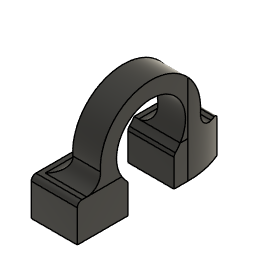
56b14100-354a-432f-bf98-abde912a1bf3 (Autodesk Fusion 360 design; units mm, degrees)
Autodesk Fusion 360 part; units mm, degrees
sketch "Esboço1" plane through (0, 0, -10.4303) normal (0, 0, 1) x (-1, 0, 0)
  line L0 (29.155, -19.6424) -> (-29.155, -19.6424)
  line L1 (-29.155, -19.6424) -> (-29.155, 12.3576)
  line L2 (-29.155, 12.3576) -> (29.155, 12.3576)
  line L3 (29.155, 12.3576) -> (29.155, -19.6424)
  circle A0 centre (-25.5, 38.3576) radius 3.95
  line L4 (15.7, 44.8576) -> (15.7, 39.0576)
  line L5 (15.7, 39.0576) -> (-15.7, 39.0576)
  line L6 (-15.7, 39.0576) -> (-15.7, 44.8576)
  line L7 (-15.7, 44.8576) -> (15.7, 44.8576)
  circle A1 centre (25.5, 38.3576) radius 3.95
  line L8 (11.25, -25.6424) -> (12.25, -26.6424)
  line L9 (12.25, -26.6424) -> (12.25, -34.1424)
  line L10 (12.25, -34.1424) -> (9.75, -34.1424)
  line L11 (9.75, -34.1424) -> (9.75, -45.1424)
  line L12 (9.75, -45.1424) -> (12.25, -45.1424)
  line L13 (12.25, -45.1424) -> (12.25, -52.6424)
  line L14 (12.25, -52.6424) -> (11.25, -53.6424)
  line L15 (11.25, -53.6424) -> (18, -53.6424)
  arc A2 (18, -53.6424) -> (28, -43.6424) centre (18, -43.6424) ccw
  line L16 (28, -43.6424) -> (28, -25.6424)
  line L17 (28, -25.6424) -> (38.8944, -20.1952)
  arc A3 (38.8944, -20.1952) -> (40, -18.4064) centre (38, -18.4064) ccw
  line L18 (40, -18.4064) -> (40, 11.1215)
  arc A4 (40, 11.1215) -> (38.8944, 12.9103) centre (38, 11.1215) ccw
  line L19 (38.8944, 12.9103) -> (32.2111, 16.252)
  arc A5 (32.2111, 16.252) -> (30.8695, 16.5687) centre (30.8695, 13.5687) ccw
  line L20 (30.8695, 16.5687) -> (28.9711, 16.5687)
  arc A6 (27.2503, 17.1112) -> (28.9711, 16.5687) centre (28.9711, 19.5687) ccw
  line L21 (27.2503, 17.1112) -> (22.237, 20.6216)
  arc A7 (21.5003, 24.7998) -> (22.237, 20.6216) centre (23.9577, 23.0791) ccw
  line L22 (21.5003, 24.7998) -> (29.1862, 35.7765)
  arc A8 (29.1862, 35.7765) -> (27.6041, 42.3354) centre (25.5, 38.3576) ccw
  line L23 (27.6041, 42.3354) -> (20.6582, 46.0094)
  arc A9 (20.6582, 46.0094) -> (19.2554, 46.3576) centre (19.2554, 43.3576) ccw
  line L24 (19.2554, 46.3576) -> (-19.2554, 46.3576)
  arc A10 (-19.2554, 46.3576) -> (-20.6582, 46.0094) centre (-19.2554, 43.3576) ccw
  line L25 (-20.6582, 46.0094) -> (-27.6041, 42.3354)
  arc A11 (-27.6041, 42.3354) -> (-29.1862, 35.7765) centre (-25.5, 38.3576) ccw
  line L26 (-29.1862, 35.7765) -> (-21.5003, 24.7998)
  arc A12 (-22.237, 20.6216) -> (-21.5003, 24.7998) centre (-23.9577, 23.0791) ccw
  line L27 (-22.237, 20.6216) -> (-27.2503, 17.1112)
  arc A13 (-28.9711, 16.5687) -> (-27.2503, 17.1112) centre (-28.9711, 19.5687) ccw
  line L28 (-28.9711, 16.5687) -> (-30.8695, 16.5687)
  arc A14 (-30.8695, 16.5687) -> (-32.2111, 16.252) centre (-30.8695, 13.5687) ccw
  line L29 (-32.2111, 16.252) -> (-38.8944, 12.9103)
  arc A15 (-38.8944, 12.9103) -> (-40, 11.1215) centre (-38, 11.1215) ccw
  line L30 (-40, 11.1215) -> (-40, -18.4064)
  arc A16 (-40, -18.4064) -> (-38.8944, -20.1952) centre (-38, -18.4064) ccw
  line L31 (-38.8944, -20.1952) -> (-28, -25.6424)
  line L32 (-28, -25.6424) -> (-28, -43.6424)
  arc A17 (-28, -43.6424) -> (-18, -53.6424) centre (-18, -43.6424) ccw
  line L33 (-18, -53.6424) -> (-11.25, -53.6424)
  line L34 (-11.25, -53.6424) -> (-12.25, -52.6424)
  line L35 (-12.25, -52.6424) -> (-12.25, -45.1424)
  line L36 (-12.25, -45.1424) -> (-9.75, -45.1424)
  line L37 (-9.75, -45.1424) -> (-9.75, -34.1424)
  line L38 (-9.75, -34.1424) -> (-12.25, -34.1424)
  line L39 (-12.25, -34.1424) -> (-12.25, -26.6424)
  line L40 (-12.25, -26.6424) -> (-11.25, -25.6424)
  line L41 (-11.25, -25.6424) -> (11.25, -25.6424)
  line L42 (-28, -31.6424) -> (-23, -31.6424)
  line L43 (-23, -31.6424) -> (-23, -47.6424)
  line L44 (-23, -47.6424) -> (-28, -47.6424)
  line L45 (-28, -47.6424) -> (-28, -31.6424)
  line L46 (-23, -39.6424) -> (-28, -39.6424) construction
  line L47 (-28, -41.6424) -> (-23, -41.6424)
  line L48 (-28, -37.6424) -> (-23, -37.6424)
  line L49 (-28, -31.6424, 0) -> (-28, -31.6424, 3.5)
  line L50 (-28, -47.6424, 3.5) -> (-28, -47.6424, 0)
  line L51 (-28, -39.6424, 0) -> (-28, -39.6424, 12) construction
  line L52 (-28, -31.6424, 0) -> (-28, -31.6424, 2.5)
  arc A18 through (-28, -34.1565, 5.6071) (-28, -39.6424, 11.5) (-28, -45.1284, 5.6071)
  line L53 (-28, -46.6246, 4) -> (-28, -47.1424, 4)
  line L54 (-28, -32.1424, 4) -> (-28, -32.6603, 4)
  arc A19 through (-28, -34.1565, 5.6071) (-28, -33.7582, 4.4779) (-28, -32.6603, 4)
  arc A20 through (-28, -45.1284, 5.6071) (-28, -45.5267, 4.4779) (-28, -46.6246, 4)
  arc A21 through (-28, -31.6424, 3.5) (-28, -31.7889, 3.8536) (-28, -32.1424, 4)
  arc A22 through (-28, -47.6424, 3.5) (-28, -47.496, 3.8536) (-28, -47.1424, 4)
  line L55 (-28, -37.1424, 0) -> (-28, -37.1424, 2.9896)
  line L56 (-28, -42.1424, 0) -> (-28, -42.1424, 2.9896)
  arc A23 through (-28, -36.9954, 3.3438) (-28, -39.6424, 9.75) (-28, -42.2895, 3.3438)
  arc A24 through (-28, -36.9954, 3.3438) (-28, -37.1042, 3.1813) (-28, -37.1424, 2.9896)
  arc A25 through (-28, -42.2895, 3.3438) (-28, -42.1807, 3.1813) (-28, -42.1424, 2.9896)
  line L57 (-28, -32.1424, 4) -> (-28, -36.4703, 4)
  line L58 (-28, -42.8146, 4) -> (-28, -47.1424, 4)
  line L59 (-23, -44.6424) -> (-28, -44.6424) construction
  line L60 (-23, -34.6424) -> (-28, -34.6424) construction
  circle A26 centre (-25.5, -34.6424) radius 1
  circle A27 centre (-25.5, -44.6424) radius 1
  dimension "d199" = 2
  dimension "d200" = 2
  dimension "d201" = 8
  dimension "d202" = 8
  dimension "d205" = 6
  dimension "d206" = 7.5
  dimension "d207" = 2.5
  dimension "d208" = 11
  dimension "d209" = 1.5
  dimension "d210" = 0.5
  dimension "d211" = 2.5
  dimension "d212" = 2.5
  dimension "d213" = 0.5
  dimension "d222" = 5
  dimension "d223" = 5
  dimension "d225" = 2
  dimension "d228" = 4
  constraint horizontal L42
  constraint vertical L43
  constraint horizontal L44
  constraint vertical L45
  constraint coincident L32 L42.start
  constraint coincident L32 L46.end
  constraint perpendicular L32 L46
  constraint coincident L43 L46.start
  constraint coincident L45 L47.start
  constraint coincident L43 L47.end
  constraint perpendicular L43 L47
  constraint coincident L45 L48.start
  constraint coincident L43 L48.end
  constraint perpendicular L43 L48
  constraint coincident L43 L59.start
  constraint coincident L45 L59.end
  constraint perpendicular L45 L59
  constraint coincident L43 L60.start
  constraint coincident L45 L60.end
  constraint parallel L48 L60
  constraint midpoint L60 A26.centre
  constraint midpoint L59 A27.centre
  constraint equal A26 A27
  measures "d199" distance of L46 L47
  measures "d200" distance of L46 L48
  measures "d201" distance of L42 L46
  measures "d202" distance of L44 L46
  measures "d205" distance of L45 L46.end
  measures "d207" distance of L42.start L45.end
  measures "d222" distance of L46 L59
  measures "d223" distance of L46 L60
  measures "d225" diameter of A27
extrude "Extrusão1" add sketch "Esboço1" along normal blind 5 contours L32 L45 L49 L52 L54 A21 L55 A23 A24 L57 | L32 L45 L50 L53 A22 L56 A23 A25 L58 in plane through (28, 0, -10.4303) normal (-1, 0, 0) makes body 1 at (26.3333, 33.4758, -10.4303) makes body 2 at (26.3333, 43.9758, -10.4303)
extrude "Extrusão2" add sketch "Esboço1" along normal blind 3 contours A18 A19 A20 A23 L57 L58 in plane through (28, 0, -10.4303) normal (-1, 0, 0) bodies 1 2
fillet "Arredondamento1" radius 1.5 2 edges at (25, 34.5653, -6.4303) (25, 44.7196, -6.4303) on bodies 1
extrude "Extrusão3" cut sketch "Esboço1" along normal blind 1 contours A26 | A27 bodies 1
extrude "Extrusão4" cut sketch "Esboço1" along normal blind 9.803 contours A17 L44 L45 bodies 1
